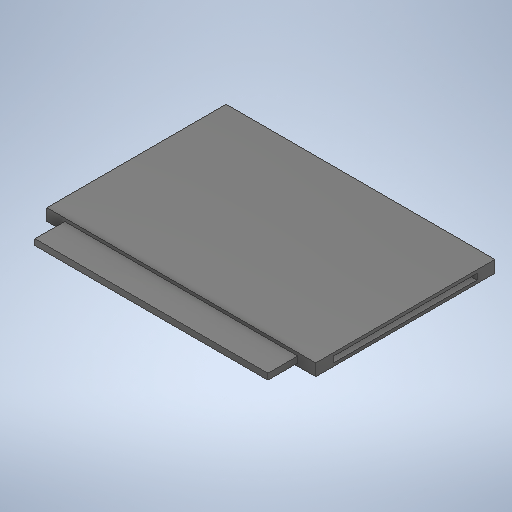
# Autodesk Inventor part: TSU_MF_Floor
Saved by Autodesk Inventor 2025.2 (Build 292293000, 293)
## iProperties
Created: 2025-01-07
Part Number: TSU_MF_Floor
Material: Generic
Document SubType Name: Modeling
Designer: Matt Tidd
Density: 1 g/cm^3
Appearance: Default
Author: Matt Tidd
Autodesk Inventor part; units mm, degrees
ref_plane "YZ Plane" through (0, 0, 0) normal (1, 0, 0) x (0, 1, 0)
ref_plane "XZ Plane" through (0, 0, 0) normal (0, 1, 0) x (-1, 0, 0)
ref_plane "XY Plane" through (0, 0, 0) normal (0, 0, 1) x (1, 0, 0)
sketch "Sketch1" plane through (0, 0, 0) normal (0, 1, 0) x (-1, 0, 0)
  line L0 (0, 0) -> (225, 0)
  line L1 (225, 0) -> (225, -150)
  line L2 (225, -150) -> (0, -150)
  line L3 (0, -150) -> (0, 0)
  dimension "d0" = 225
  dimension "d1" = 150
  constraints: 8 end point, 2 parallel, 1 horizontal, 1 perpendicular
  measures "d0" distance of L1.end L2.end
  measures "d1" distance of L0.end L1.end
extrude "Extrusion1" add sketch "Sketch1" along normal blind 10
sketch "Sketch2" plane through (-225, 0, 0) normal (0, 0, 1) x (1, 0, 0)
  line L0 (0, 0) -> (0, 10) projected
  line L1 (225, 0) -> (225, 10) projected
  line L2 (0, 7.5) -> (225, 7.5)
  line L3 (225, 7.5) -> (225, 2.5)
  line L4 (225, 2.5) -> (0, 2.5)
  line L5 (0, 2.5) -> (0, 7.5)
  line L6 (225, 7.5) -> (210, 7.5)
  line L7 (210, 7.5) -> (210, 2.5)
  line L8 (210, 2.5) -> (225, 2.5)
  line L9 (225, 2.5) -> (225, 7.5)
  line L10 (0, 7.5) -> (15, 7.5)
  line L11 (15, 7.5) -> (15, 2.5)
  line L12 (15, 2.5) -> (0, 2.5)
  line L13 (0, 2.5) -> (0, 7.5)
  dimension "d4" = 5
  dimension "d5" = 15
  dimension "d6" = 5
  dimension "d7" = 15
  dimension "d8" = 5
  constraints: 24 end point, 6 parallel, 3 horizontal, 3 perpendicular, 2 point on line
  measures "d4" distance of L2.end L3.end
  measures "d5" distance of L8.end L7.end
  measures "d6" distance of L7.end L6.end
  measures "d7" distance of L11.end L12.end
  measures "d8" distance of L10.end L11.end
sketch "Sketch3" plane through (0, 0, 0) normal (1, 0, 0) x (0, 0, -1)
  line L0 (0, 0) -> (0, 10) projected
  line L1 (0, 7.5) -> (150, 7.5)
  line L2 (150, 7.5) -> (150, 2.5)
  line L3 (150, 2.5) -> (0, 2.5)
  line L4 (0, 2.5) -> (0, 7.5)
  line L5 (0, 7.5) -> (15, 7.5)
  line L6 (15, 7.5) -> (15, 2.5)
  line L7 (15, 2.5) -> (0, 2.5)
  line L8 (0, 2.5) -> (0, 7.5)
  line L9 (150, 7.5) -> (135, 7.5)
  line L10 (135, 7.5) -> (135, 2.5)
  line L11 (135, 2.5) -> (150, 2.5)
  line L12 (150, 2.5) -> (150, 7.5)
  dimension "d9" = 150
  dimension "d10" = 5
  dimension "d11" = 15
  dimension "d12" = 5
  dimension "d13" = 15
  dimension "d14" = 5
  constraints: 24 end point, 6 parallel, 3 horizontal, 3 perpendicular, 1 point on line
  measures "d9" distance of L2.end L3.end
  measures "d10" distance of L1.end L2.end
  measures "d11" distance of L6.end L7.end
  measures "d12" distance of L5.end L6.end
  measures "d13" distance of L11.end L10.end
  measures "d14" distance of L10.end L9.end
extrude "Extrusion2" add sketch "Sketch2" along normal blind 25 contours L11 L2 L7 L4
extrude "Extrusion3" cut sketch "Sketch3" against normal blind 25 contours L6 L1 L10 L3
sketch "Sketch4" plane through (0, 0, 0) normal (0, -1, 0) x (1, 0, 0)
  line L0 (-225, -150) -> (-225, 0) projected
  line L1 (-225, -50) -> (-215, -50)
  line L2 (-215, -50) -> (-215, -80)
  line L3 (-215, -80) -> (-225, -80)
  line L4 (-225, -80) -> (-225, -50)
  line L5 (-50, -150) -> (-155, -150)
  line L6 (-155, -150) -> (-155, -140)
  line L7 (-155, -140) -> (-50, -140)
  line L8 (-50, -140) -> (-50, -150)
  point P0 (0, 0)
  dimension "d19" = 10
  dimension "d20" = 30
  dimension "d21" = 105
  dimension "d22" = 10
  constraints: 16 end point, 4 parallel, 2 horizontal, 2 perpendicular, 1 point on line
  measures "d19" distance of L2.end L3.end
  measures "d20" distance of L1.end L2.end
  measures "d21" distance of L6.end L7.end
  measures "d22" distance of L5.end L6.end
extrude "Extrusion4" add sketch "Sketch4" along normal blind 10
body "Solid1"
